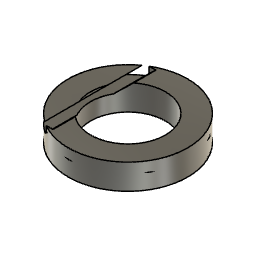
Mirror Mount- New Version v3 (Autodesk Fusion 360 design; units mm, degrees)
Autodesk Fusion 360 part; units mm, degrees
sketch "Sketch1" plane through (0, 0, 0) normal (0, 0, 1) x (1, 0, 0)
  circle A0 centre (0, 0) radius 22.225
  circle A1 centre (0, 0) radius 35.425
  circle A2 centre (0, 29.3625) radius 6
  circle A3 centre (-25.4287, 14.6813) radius 6
  circle A4 centre (-25.4287, -14.6812) radius 6
  circle A5 centre (0, -29.3625) radius 6
  circle A6 centre (25.4287, -14.6813) radius 6
  circle A7 centre (25.4287, 14.6812) radius 6
  dimension "d1" = 44.45
  dimension "d2" = 70.85
  dimension "d3" = 12
  dimension "d4" = 29.3625
  dimension "d6" = 360
  constraint coincident A0.centre A1.centre
  constraint concentric A0 A1
  constraint vertical A0.centre A2.centre
  measures "d1" diameter of A0
  measures "d2" diameter of A1
  measures "d3" diameter of A2
  measures "d4" vertical distance of A0.centre A2.centre
extrude "Extrude1" add sketch "Sketch1" along normal blind 15 contours A1 | A2 | A3 | A4 | A5 | A6 | A7 makes body 1
extrude "Extrude2" cut sketch "Sketch1" along normal blind 9 contours A2 | A3 | A4 | A5 | A6 | A7 bodies 1
sketch "Sketch2" plane through (0, 0, 0) normal (0, 1, 0) x (1, 0, 0)
  line L0 (-15.955, -19.2911) -> (-26, -9.924)
  line L1 (-26, -9.924) -> (-19.4017, -9.924)
  line L2 (-19.4017, -9.924) -> (-12.886, -16)
  line L3 (-12.886, -16) -> (-15.955, -19.2911)
  line L4 (0, 0) -> (0, -30.1801) construction
  line L5 (-35.425, -15) -> (35.425, -15)
  dimension "d11" = 47
  dimension "d12" = 4.5
  dimension "d13" = 5.076
  dimension "d14" = 26
  dimension "d15" = 1
  constraint coincident L4.start origin
  constraint vertical L4
  constraint horizontal L1
  constraint parallel L0 L2
  constraint perpendicular L0 L3
  measures "d11" angle of L2 L4
  measures "d12" distance of L0.start L2.end
  measures "d13" distance of L1 L5
  measures "d14" distance of L0.end L4
  measures "d15" distance of L2.end L5
extrude "Extrude3" cut sketch "Sketch2" along normal mid plane 61 bodies 1
copy_body "Body->Comp1" bodies 1 removing the originals makes body 2 in component "Component"
sketch "Sketch3" plane through (0, 0, 0) normal (0, 1, 0) x (1, 0, 0)
  line L0 (0, -15) -> (50, -4)
  line L1 (50, -4) -> (50, -15)
  line L2 (0, -15) -> (50, -15)
  line L3 (-18.0189, -15) -> (35.425, -15)
  dimension "d19" = 50
  dimension "d25" = 11
  constraint vertical L1
  constraint horizontal L2
  constraint vertical origin L0.start
  constraint coincident L0.start L3
  measures "d19" distance of origin L1
  measures "d25" distance of L0.end L1.end
component "Component" placed x (1, 0, 0) y (0, 1, 0) z (0, 0, 1) at (0, 0, 0)
